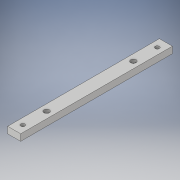
# Autodesk Inventor part: RioConnectors
Saved by Autodesk Inventor 2019 (Build 230136000, 136)
## iProperties
Created: 2018-12-25
Part Number: RioConnectors
Material: Generic
Document SubType Name: Modeling
Designer: james
Density: 1 g/cm^3
Appearance: Default
Author: james
Autodesk Inventor part; units mm, degrees
ref_plane "YZ Plane" through (0, 0, 0) normal (1, 0, 0) x (0, 1, 0)
ref_plane "XZ Plane" through (0, 0, 0) normal (0, 1, 0) x (-1, 0, 0)
ref_plane "XY Plane" through (0, 0, 0) normal (0, 0, 1) x (1, 0, 0)
sketch "Sketch1" plane through (0, 0, 0) normal (0, 1, 0) x (-1, 0, 0)
  line L0 (23.1483, 102.1323) -> (7.9083, 102.1323)
  line L1 (7.9083, 102.1323) -> (7.9083, -75.6677)
  line L2 (7.9083, -75.6677) -> (23.1483, -75.6677)
  line L3 (23.1483, -75.6677) -> (23.1483, 102.1323)
  point P0 (0, 0)
  dimension "d0" = 177.8
  dimension "d1" = 15.24
  constraints: 8 end point, 2 parallel, 1 horizontal, 1 perpendicular
  measures "d0" distance of L2.end L0.start
  measures "d1" distance of L0.start L0.end
extrude "Extrusion1" add sketch "Sketch1" along normal blind 7.62
sketch "Sketch2" plane through (0, 7.62, 0) normal (0, 1, 0) x (1, 0, 0)
  line L0 (-23.1483, 75.6677) -> (-23.1483, -102.1323) projected
  line L1 (-7.9083, 75.6677) -> (-23.1483, 75.6677) projected
  line L2 (-23.1483, -102.1323) -> (-7.9083, -102.1323) projected
  point P0 (0, 0)
  point P1 (-15.5283, -64.0323)
  point P2 (-15.5283, 37.5677)
  dimension "d4" = 0
  dimension "d5" = 101.6
  dimension "d6" = 7.62
  dimension "d7" = 38.1
  dimension "d8" = 38.1
  measures "d4" horizontal distance of point (-15.528, -64.032) point (-15.528, 37.568)
  measures "d5" distance of point (-15.528, -64.032) point (-15.528, 37.568)
  measures "d6" distance from line of L0 point (-15.528, 37.568)
  measures "d7" distance from line of L1 point (-15.528, 37.568)
  measures "d8" distance from line of L2 point (-15.528, -64.032)
hole "Hole1" at (-15.5283, 7.62, 64.0323) at (-15.5283, 7.62, -37.5677) direction (0, -1, 0) diameter 2.794 end through all
sketch "Sketch3" plane through (0, 7.62, 0) normal (0, 1, 0) x (1, 0, 0)
  circle A0 centre (-15.5283, -64.0323) radius 1.397 projected
  circle A1 centre (-15.5283, 37.5677) radius 1.397 projected
  circle A2 centre (-15.5283, -64.0323) radius 3.175
  circle A3 centre (-15.5283, 37.5677) radius 3.175
  point P0 (0, 0)
  dimension "d16" = 6.35
  dimension "d17" = 6.35
  constraints: 2 centre point, 2 coincident
  measures "d16" diameter of A2
  measures "d17" diameter of A3
extrude "Extrusion2" cut sketch "Sketch3" against normal blind 3.048
sketch "Sketch4" plane through (0, 7.62, 0) normal (0, 1, 0) x (1, 0, 0)
  line L0 (-7.9083, -102.1323) -> (-7.9083, 75.6677) projected
  line L1 (-23.1483, -102.1323) -> (-7.9083, -102.1323) projected
  line L2 (-7.9083, 75.6677) -> (-23.1483, 75.6677) projected
  point P0 (0, 0)
  point P1 (-15.5283, -91.9723)
  point P2 (-15.5283, 65.5077)
  dimension "d20" = 0
  dimension "d21" = 7.62
  dimension "d22" = 10.16
  dimension "d23" = 10.16
  measures "d20" horizontal distance of point (-15.528, -91.972) point (-15.528, 65.508)
  measures "d21" distance from line of L0 point (-15.528, -91.972)
  measures "d22" distance from line of L1 point (-15.528, -91.972)
  measures "d23" distance from line of L2 point (-15.528, 65.508)
hole "Hole2" at (-15.5283, 7.62, 91.9723) at (-15.5283, 7.62, -65.5077) direction (0, -1, 0) diameter 4.826 end through all
body "Solid1"
